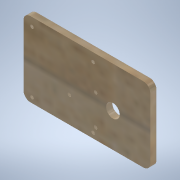
# Autodesk Inventor part: 前後直動12x12_4
Saved by Autodesk Inventor 2020.3 (Build 243373000, 373)
## iProperties
Created: 2020-07-05
Part Number: 前後直動12x12_4
Material: 木材 (カエデ材)
Document SubType Name: Modeling
Designer: totot
Density: 0.67 g/cm^3
Appearance: ナチュラル カエデ材 - 光沢 濃い着色
Mass: 15.3389 g
Surface Area: 102.906 cm^2
Volume: 22.8939 cm^3
Author: totot
Autodesk Inventor part; units mm, degrees
ref_plane "YZ Plane" through (0, 0, 0) normal (1, 0, 0) x (0, 1, 0)
ref_plane "XZ Plane" through (0, 0, 0) normal (0, 1, 0) x (-1, 0, 0)
ref_plane "XY Plane" through (0, 0, 0) normal (0, 0, 1) x (1, 0, 0)
sketch "スケッチ1" plane through (0, 0, 0) normal (0, 0, 1) x (1, 0, 0)
  line L0 (0, 0) -> (112, 0)
  line L1 (112, 0) -> (112, -75)
  line L2 (112, -75) -> (0, -75)
  line L3 (0, -75) -> (0, 0)
  dimension "d0" = 112
  dimension "d1" = 75
  constraints: 8 end point, 2 parallel, 1 horizontal, 1 perpendicular
  measures "d0" distance of L1.end L2.end
  measures "d1" distance of L0.end L1.end
extrude "押し出し1" add sketch "スケッチ1" along normal blind 5.5
sketch "スケッチ2" plane through (0, 0, 5.5) normal (0, 0, 1) x (1, 0, 0)
  line L0 (112, 0) -> (0, 0) projected
  line L1 (0, 0) -> (0, -75) projected
  line L2 (0, -75) -> (112, -75) projected
  point P0 (7.5, -7.5)
  point P1 (107.5, -7.5)
  point P2 (107.5, -67.5)
  point P3 (7.5, -67.5)
  dimension "d4" = 7.5
  dimension "d5" = 7.5
  dimension "d6" = 7.5
  dimension "d7" = 100
  dimension "d8" = 60
  dimension "d9" = 60
  dimension "d10" = 100
  dimension "d19" = 7.5
  dimension "d51" = 7.5
  measures "d4" distance from line of point (7.5, -7.5) L0
  measures "d5" distance from line of point (7.5, -7.5) L1
  measures "d6" distance from line of L0 point (107.5, -7.5)
  measures "d7" distance of point (107.5, -7.5) point (7.5, -7.5)
  measures "d8" distance of point (7.5, -67.5) point (7.5, -7.5)
  measures "d9" distance of point (107.5, -7.5) point (107.5, -67.5)
  measures "d10" distance of point (7.5, -67.5) point (107.5, -67.5)
  measures "d19" distance from line of L1 point (7.5, -67.5)
  measures "d51" distance from line of L2 point (7.5, -67.5)
hole "穴1" at (7.5, -7.5, 5.5) at (107.5, -7.5, 5.5) at (107.5, -67.5, 5.5) at (7.5, -67.5, 5.5) direction (0, 0, -1) diameter 3 end through all
fillet "フィレット1" radius 6 4 edges at (112, 0, 2.75) (112, -75, 2.75) (0, 0, 2.75) (0, -75, 2.75)
sketch "スケッチ3" plane through (0, 0, 0) normal (0, 0, -1) x (-1, 0, 0)
  circle A0 centre (-42, -45) radius 15.5
  line L0 (-112, -69) -> (-112, -6) projected
  line L1 (0, -6) -> (0, -69) projected
  line L2 (-106, 0) -> (-6, 0) projected
  line L3 (-6, -75) -> (-106, -75) projected
  line L4 (-42, -45) -> (-26.5, -45)
  line L5 (-42, -45) -> (-49.75, -31.5766)
  line L6 (-42, -45) -> (-49.75, -58.4234)
  point P0 (0, 0)
  dimension "d20" = 31
  dimension "d21" = 70
  dimension "d22" = 112
  dimension "d23" = 75
  dimension "d24" = 30
  dimension "d25" = 120
  dimension "d26" = 120
  constraints: 6 end point, 3 coincident, 3 point on circle, 1 centre point, 1 horizontal
  measures "d20" diameter of A0
  measures "d21" distance from line of L4.start L0
  measures "d22" distance between parallel lines of L0 L1
  measures "d23" distance between parallel lines of L2 L3
  measures "d24" distance from line of L4.start L3
  measures "d25" angle of L5 L4
  measures "d26" angle of L5 L6
hole "穴2" at (49.75, -58.4234, 0) at (49.75, -31.5766, 0) at (26.5, -45, 0) direction (0, 0, 1) diameter 3 end through all
sketch "スケッチ4" plane through (0, 0, 0) normal (0, 0, -1) x (-1, 0, 0)
  line L0 (-42, -45) -> (-42, -38)
  line L1 (-6, -75) -> (-106, -75) projected
  line L2 (-106, 0) -> (-6, 0) projected
  line L3 (-112, -69) -> (-112, -6) projected
  point P0 (0, 0)
  dimension "d34" = 7
  dimension "d35" = 30
  dimension "d36" = 75
  dimension "d37" = 70
  constraints: 2 end point, 1 coincident, 1 vertical
  measures "d34" distance of L0.start L0.end
  measures "d35" distance from line of L0.start L1
  measures "d36" distance between parallel lines of L2 L1
  measures "d37" distance between parallel lines of L0 L3
hole "穴3" at (42, -38, 0) direction (0, 0, 1) diameter 12 end through all
sketch "スケッチ5" plane through (0, 0, 5.5) normal (0, 0, 1) x (1, 0, 0)
  circle A0 centre (72, -38) radius 4
  circle A1 centre (42, -38) radius 6 projected
  line L0 (106, 0) -> (6, 0) projected
  point P0 (0, 0)
  dimension "d45" = 8
  dimension "d46" = 30
  dimension "d47" = 38
  dimension "d48" = 38
  constraints: 1 centre point
  measures "d45" diameter of A0
  measures "d46" distance of A0.centre A1.centre
  measures "d47" distance from line of A1.centre L0
  measures "d48" distance from line of A0.centre L0
extrude "押し出し2" cut sketch "スケッチ5" against normal through all contours A0
equation "\"d4\" = d5"
equation "\"d5\" = d19"
equation "\"d6\" = d4"
equation "\"d9\" = d8"
equation "\"d10\" = d7"
equation "\"d48\" = d47"
